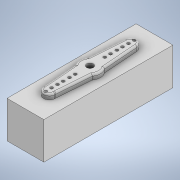
# Autodesk Inventor part: Large to Small horn Adapter
Saved by Autodesk Inventor 2020 (Build 240168000, 168)
## iProperties
Created: 2020-04-13
Part Number: Large to Small horn Adapter
Material: Generic
Document SubType Name: Modeling
Designer: varun
Density: 1 g/cm^3
Appearance: Default
Author: varun
Autodesk Inventor part; units mm, degrees
ref_plane "YZ Plane" through (0, 0, 0) normal (1, 0, 0) x (0, 1, 0)
ref_plane "XZ Plane" through (0, 0, 0) normal (0, 1, 0) x (-1, 0, 0)
ref_plane "XY Plane" through (0, 0, 0) normal (0, 0, 1) x (1, 0, 0)
sketch "Sketch1" plane through (0, 0, 0) normal (0, 1, 0) x (-1, 0, 0)
  line L0 (-6.35, 22.225) -> (6.35, 22.225)
  line L1 (6.35, 22.225) -> (6.35, -22.225)
  line L2 (6.35, -22.225) -> (-6.35, -22.225)
  line L3 (-6.35, -22.225) -> (-6.35, 22.225)
  line L4 (-6.35, 22.225) -> (6.35, -22.225) construction
  line L5 (6.35, 22.225) -> (-6.35, -22.225) construction
  point P0 (0, 0)
  dimension "d0" = 12.7
  dimension "d1" = 44.45
  constraints: 12 end point, 2 midpoint, 2 parallel, 1 horizontal, 1 perpendicular
  measures "d0" distance of L1.end L2.end
  measures "d1" distance of L0.end L1.end
extrude "Extrusion1" add sketch "Sketch1" along normal blind 12.7
sketch "Sketch2" plane through (0, 12.7, 0) normal (0, 1, 0) x (1, 0, 0)
  circle A0 centre (0, 0) radius 1.15
  circle A1 centre (0, -7.0718) radius 0.5
  circle A2 centre (0, -9.2663) radius 0.5
  circle A3 centre (0, -11.1889) radius 0.5
  circle A4 centre (0, -13.2339) radius 0.5
  circle A5 centre (0, -15.222) radius 0.5
  circle A6 centre (0, -5.0783) radius 0.5
  line L0 (0, 0) -> (3.58, 0)
  circle A7 centre (0, 0) radius 1.15
  circle A8 centre (0, 7.0718) radius 0.5
  circle A9 centre (0, 9.2663) radius 0.5
  circle A10 centre (0, 11.1889) radius 0.5
  circle A11 centre (0, 13.2339) radius 0.5
  circle A12 centre (0, 15.222) radius 0.5
  circle A13 centre (0, 5.0783) radius 0.5
  circle A14 centre (0, 0) radius 3.58
  line L1 (-2.875, 2.1333) -> (-1.9947, 14.1462)
  line L2 (1.9947, 14.1462) -> (2.875, 2.1333)
  line L3 (2.875, -2.1333) -> (1.9947, -13.7339)
  line L4 (-1.9947, -14.1462) -> (-2.875, -2.1333)
  arc A15 (1.9947, 14.1462) -> (-1.9947, 14.1462) centre (0, 14) ccw
  arc A16 (-1.9947, -14.1462) -> (1.9947, -14.1462) centre (0, -14) ccw
  circle A17 centre (0, 0) radius 3.58
  line L5 (1.9947, -14.1462) -> (1.9947, -13.7339)
  constraints: 18 centre point, 12 end point, 6 symmetric about line, 4 point on circle, 1 horizontal, 1 vertical, 7 other
extrude "Extrusion2" add sketch "Sketch2" along normal blind 1.778
fillet "Fillet1" radius 0.635 9 edges at (1.9947, 14.478, 13.94) (2.4348, 14.478, 7.9336) (-2.4348, 14.478, 8.1397) (0, 14.478, 16) (3.58, 14.478, 0) (0, 14.478, -16) (-2.4348, 14.478, -8.1397) (2.4348, 14.478, -8.1397) (-3.58, 14.478, 0)
body "Solid1"
